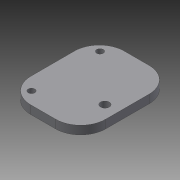
# Autodesk Inventor part: Carriage_Frame_Back
Saved by Autodesk Inventor 2014 (Build 180170000, 170)
## iProperties
Created: 2014-08-27
Part Number: Carriage_Frame_Back
Material: Generic
Document SubType Name: Modeling
Designer: ThatOtherGuy
Density: 1 g/cm^3
Appearance: Default
Author: ThatOtherGuy
Autodesk Inventor part; units mm, degrees
ref_plane "YZ Plane" through (0, 0, 0) normal (1, 0, 0) x (0, 1, 0)
ref_plane "XZ Plane" through (0, 0, 0) normal (0, 1, 0) x (-1, 0, 0)
ref_plane "XY Plane" through (0, 0, 0) normal (0, 0, 1) x (1, 0, 0)
sketch "Sketch1" plane through (0, 0, 0) normal (0, 0, 1) x (1, 0, 0)
  circle A0 centre (10.5, 65) radius 2.65
  circle A1 centre (10.5, 10) radius 2.65
  circle A2 centre (49.5, 30) radius 3.5
  line L0 (0, 0) -> (60, 0)
  line L1 (60, 0) -> (60, 75)
  line L2 (60, 75) -> (0, 75)
  line L3 (0, 75) -> (0, 0)
  dimension "d0" = 39
  dimension "d1" = 5.3
  dimension "d2" = 55
  dimension "d16" = 7
  dimension "d26" = 75
  dimension "d27" = 60
  dimension "d28" = 10
  dimension "d29" = 10.5
  dimension "d32" = 20
  dimension "d44" = 10.5
  dimension "d50" = 10
  constraints: 12 end point, 3 centre point, 2 parallel, 1 coincident, 1 equal radius, 1 horizontal, 1 perpendicular, 1 vertical alignment
  measures "d0" horizontal distance of A0.centre A2.centre
  measures "d1" diameter of A0
  measures "d2" distance of A0.centre A1.centre
  measures "d16" diameter of A2
  measures "d26" distance between parallel lines of L0 L2
  measures "d27" distance between parallel lines of L3 L1
  measures "d28" distance from line of L0 A1.centre
  measures "d29" distance from line of L3 A1.centre
  measures "d32" vertical distance of A2.centre A1.centre
  measures "d44" distance from line of L1 A2.centre
  measures "d50" distance from line of L2 A0.centre
extrude "Extrusion1" add sketch "Sketch1" along normal blind 6.731
fillet "Fillet1" radius 20 4 edges at (0, 75, 3.3655) (60, 75, 3.3655) (0, 0, 3.3655) (60, 0, 3.3655)
equation "\"d29\" = d44"
equation "\"d30\" = THICKB"
equation "\"THICKA\" = 3.175"
equation "\"THICKB\" = 6.731"
equation "\"THICKC\" = 12.7"
equation "\"BALLDIA\" = 12"
equation "\"MAGDIA\" = 9.5"
equation "\"THICKPLY\" = 5"
body "Solid1"
